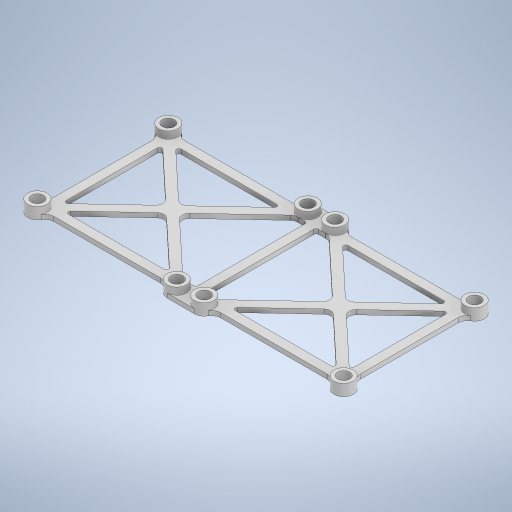
# Autodesk Inventor part: Display_Standof_2.5
Saved by Autodesk Inventor 2023 (Build 270158000, 158)
## iProperties
Created: 2023-02-18
Part Number: Display_Standof_2.5
Material: Generisch
Document SubType Name: Modeling
Designer: dvd62
Density: 1 g/cm^3
Appearance: Vorgabe
Author: dvd62
Autodesk Inventor part; units mm, degrees
ref_plane "YZ Plane" through (0, 0, 0) normal (1, 0, 0) x (0, 1, 0)
ref_plane "XZ Plane" through (0, 0, 0) normal (0, 1, 0) x (-1, 0, 0)
ref_plane "XY Plane" through (0, 0, 0) normal (0, 0, 1) x (1, 0, 0)
sketch "Skizze1" plane through (0, 0, 0) normal (0, 1, 0) x (-1, 0, 0)
  circle A0 centre (0, 0) radius 1.35
  circle A1 centre (-30.8, 0) radius 1.35
  circle A2 centre (-36.83, 0) radius 1.35
  circle A3 centre (-67.63, 0) radius 1.35
  circle A4 centre (0, -28.9) radius 1.35
  circle A5 centre (-30.8, -28.9) radius 1.35
  circle A6 centre (-36.83, -28.9) radius 1.35
  circle A7 centre (-67.63, -28.9) radius 1.35
  line L0 (0, 0) -> (-67.63, 0) construction
  line L1 (-67.63, 0) -> (-67.63, -28.9) construction
  line L2 (-67.63, -28.9) -> (0, -28.9) construction
  line L3 (0, -28.9) -> (0, 0) construction
  circle A8 centre (0, -28.9) radius 2.15
  circle A9 centre (-30.8, -28.9) radius 2.15
  circle A10 centre (-36.83, -28.9) radius 2.15
  circle A11 centre (-67.63, -28.9) radius 2.15
  circle A12 centre (-67.63, 0) radius 2.15
  circle A13 centre (-36.83, 0) radius 2.15
  circle A14 centre (-30.8, 0) radius 2.15
  circle A15 centre (0, 0) radius 2.15
  line L4 (0, -26.75) -> (0, -2.15)
  line L5 (-2.15, 0) -> (-28.65, 0)
  line L6 (-32.95, 0) -> (-34.68, 0)
  line L7 (-38.98, 0) -> (-65.48, 0)
  line L8 (-67.63, -2.15) -> (-67.63, -26.75)
  line L9 (-65.48, -28.9) -> (-38.98, -28.9)
  line L10 (-34.68, -28.9) -> (-32.95, -28.9)
  line L11 (-28.65, -28.9) -> (-2.15, -28.9)
  line L12 (-2, -2) -> (-65.63, -2)
  line L13 (-65.63, -2) -> (-65.63, -26.9)
  line L14 (-65.63, -26.9) -> (-2, -26.9)
  line L15 (-2, -26.9) -> (-2, -2)
  line L16 (0, -28.9) -> (-30.8, 0) construction
  line L17 (0, 0) -> (-30.8, -28.9) construction
  line L18 (-36.83, -28.9) -> (-67.63, 0) construction
  line L19 (-67.63, -28.9) -> (-36.83, 0) construction
  line L20 (-27.2071, -2) -> (-2, -25.6521)
  line L21 (-3.5929, -26.9) -> (-30.0963, -2.0316)
  line L22 (-2, -3.2479) -> (-27.2071, -26.9)
  line L23 (-3.5929, -2) -> (-30.0963, -26.8684)
  line L24 (-64.0371, -2) -> (-37.5337, -26.8684)
  line L25 (-65.63, -3.2479) -> (-40.4229, -26.9)
  line L26 (-37.5337, -2.0316) -> (-64.0371, -26.9)
  line L27 (-65.63, -25.6521) -> (-40.4229, -2)
  line L28 (-33.815, -2) -> (-33.815, -26.9) construction
  line L29 (-32.815, -26.9) -> (-32.815, -2)
  line L30 (-34.815, -2) -> (-34.815, -26.9)
  line L31 (-36.83, -31.05) -> (-30.8, -31.05)
  line L32 (-30.8, -26.75) -> (-36.83, -26.75)
  line L33 (-30.8, -2.15) -> (-36.83, -2.15)
  line L34 (-30.8, 2.15) -> (-36.83, 2.15)
  point P0 (-31.589, -2)
  point P1 (-16.8614, -14.45)
  point P2 (-31.589, -26.9)
  point P3 (-36.041, -26.9)
  point P4 (-50.7686, -14.45)
  point P5 (-36.041, -2)
  point P6 (-52.23, -13.0787)
  point P7 (-53.6914, -14.45)
  point P8 (-52.23, -15.8213)
  point P9 (-13.9386, -14.45)
  point P10 (-15.4, -13.0787)
  point P11 (-15.4, -15.8213)
  point P12 (-34.815, -2.15)
  point P13 (-32.815, -2.15)
  point P14 (-32.815, -26.75)
  point P15 (-34.815, -26.75)
  dimension "d0" = 2.7
  dimension "d1" = 2.7
  dimension "d2" = 2.7
  dimension "d3" = 2.7
  dimension "d4" = 2.7
  dimension "d5" = 2.7
  dimension "d7" = 2.7
  dimension "d8" = 2.7
  dimension "d9" = 30.8
  dimension "d10" = 6.03
  dimension "d11" = 30.8
  dimension "d12" = 28.9
  dimension "d13" = 30.8
  dimension "d14" = 6.03
  dimension "d15" = 30.8
  dimension "d16" = 0.8
  dimension "d17" = 0.8
  dimension "d18" = 0.8
  dimension "d19" = 0.8
  dimension "d20" = 0.8
  dimension "d21" = 0.8
  dimension "d22" = 0.8
  dimension "d23" = 0.8
  dimension "d24" = 2
  dimension "d25" = 2
  dimension "d26" = 2
  dimension "d27" = 2
  dimension "d28" = 2
  dimension "d29" = 2
  dimension "d30" = 2
  dimension "d31" = 2
  dimension "d34" = 2
  constraints: 62 end point, 28 point on circle, 16 centre point, 9 point on line, 8 parallel, 6 tangent, 4 vertical, 2 coincident, 1 horizontal, 49 other
  measures "d0" diameter of A0
  measures "d1" diameter of A1
  measures "d2" diameter of A2
  measures "d3" diameter of A3
  measures "d4" diameter of A4
  measures "d5" diameter of A5
  measures "d7" diameter of A6
  measures "d8" diameter of A7
  measures "d9" distance of L16.end point (0, 0)
  measures "d10" distance of A2.centre L16.end
  measures "d11" distance of A3.centre A2.centre
  measures "d12" distance of L3.start point (0, 0)
  measures "d13" distance of L17.end A4.centre
  measures "d14" distance of L17.end L18.start
  measures "d15" distance of L1.end L18.start
  measures "d16" radial gap between concentric circles of A4 A8
  measures "d17" radial gap between concentric circles of A5 A9
  measures "d18" radial gap between concentric circles of A6 A10
  measures "d19" radial gap between concentric circles of A7 A11
  measures "d20" radial gap between concentric circles of A3 A12
  measures "d21" radial gap between concentric circles of A2 A13
  measures "d22" radial gap between concentric circles of A1 A14
  measures "d23" radial gap between concentric circles of A0 A15
  measures "d24" distance between parallel lines of L3 L15
  measures "d26" distance between parallel lines of L8 L13
  measures "d28" distance between parallel lines of L21 L20
  measures "d29" distance between parallel lines of L22 L23
  measures "d30" distance between parallel lines of L25 L24
  measures "d31" distance between parallel lines of L26 L27
  measures "d34" distance between parallel lines of L29 L30
extrude "Extrusion1" add sketch "Skizze1" along normal blind 1 contours A8 | A8 L11 A9 L14 L15 L12 A14 L5 A15 L4 | A15 | A9 L14 | L31 A10 L10 A9 | L14 A9 | A9 L23 L21 L22 L14 | A14 L12 | L10 A10 L14 A9 | A10 L14 | L14 L29 L32 A9 | A14 L6 A13 L34 | L12 L20 L23 L21 A14 | A14 L12 | L9 A11 L8 A12 L7 A13 L12 L13 L14 A10 | L23 L20 L22 L21 | L14 L30 L32 L29 | L21 L22 L20 L15 L14 | A14 L12 A13 L6 | A13 L12 | A14 L33 L29 L12 | L14 A10 | A10 L32 L30 L14 | L14 L25 L26 L24 A10 | A11 | L32 L30 L33 L29 | L23 L12 L15 L22 L20 | L29 L33 L30 L12 | L12 L30 L33 A13 | A13 L12 | A13 L26 L24 L27 L12 | A12 | L26 L25 L27 L24 | L14 L13 L27 L25 L26 | L27 L25 L13 L12 L24
sketch "Skizze2" plane through (0, 1, 0) normal (0, 1, 0) x (1, 0, 0)
  circle A0 centre (0, 28.9) radius 1.35 projected
  arc A1 (2.15, 28.9) -> (0, 26.75) centre (0, 28.9) ccw projected
  arc A2 (38.98, 0) -> (28.65, 28.9) centre (30.8, 28.9) ccw projected
  circle A3 centre (30.8, 28.9) radius 1.35 projected
  circle A4 centre (36.83, 28.9) radius 1.35 projected
  arc A5 (38.98, 28.9) -> (38.98, 0) centre (36.83, 28.9) ccw projected
  arc A6 (67.63, 26.75) -> (65.48, 28.9) centre (67.63, 28.9) ccw projected
  circle A7 centre (67.63, 28.9) radius 1.35 projected
  circle A8 centre (67.63, 0) radius 1.35 projected
  arc A9 (65.48, 0) -> (67.63, 2.15) centre (67.63, 0) ccw projected
  arc A10 (38.98, 0) -> (38.98, 0) centre (36.83, 0) ccw projected
  arc A11 (28.65, 0) -> (38.98, 0) centre (30.8, 0) ccw projected
  circle A12 centre (30.8, 0) radius 1.35 projected
  arc A13 (0, 2.15) -> (2.15, 0) centre (0, 0) ccw projected
  circle A14 centre (0, 0) radius 1.35 projected
  arc A15 (36.83, -2.15) -> (38.98, 0) centre (36.83, 0) ccw projected
  line L0 (38.98, 0) -> (65.48, 0) projected
  arc A16 (65.48, 0) -> (67.63, 2.15) centre (67.63, 0) ccw projected
  line L1 (67.63, 2.15) -> (67.63, 26.75) projected
  arc A17 (67.63, 26.75) -> (65.48, 28.9) centre (67.63, 28.9) ccw projected
  line L2 (65.48, 28.9) -> (38.98, 28.9) projected
  arc A18 (38.98, 28.9) -> (36.83, 31.05) centre (36.83, 28.9) ccw projected
  arc A19 (30.8, 31.05) -> (28.65, 28.9) centre (30.8, 28.9) ccw projected
  line L3 (28.65, 28.9) -> (2.15, 28.9) projected
  arc A20 (2.15, 28.9) -> (0, 26.75) centre (0, 28.9) ccw projected
  line L4 (0, 26.75) -> (0, 2.15) projected
  arc A21 (0, 2.15) -> (2.15, 0) centre (0, 0) ccw projected
  line L5 (2.15, 0) -> (28.65, 0) projected
  arc A22 (28.65, 0) -> (30.8, -2.15) centre (30.8, 0) ccw projected
  line L6 (32.815, 26.75) -> (32.815, 2.15) projected
  arc A23 (30.8, 2.15) -> (30.0963, 2.0316) centre (30.8, 0) ccw projected
  line L7 (30.0963, 2.0316) -> (16.8614, 14.45) projected
  line L8 (16.8614, 14.45) -> (30.0963, 26.8684) projected
  arc A24 (30.0963, 26.8684) -> (30.8, 26.75) centre (30.8, 28.9) ccw projected
  circle A25 centre (67.63, 0) radius 1.35 projected
  circle A26 centre (67.63, 28.9) radius 1.35 projected
  circle A27 centre (36.83, 28.9) radius 1.35 projected
  line L9 (64.0371, 2) -> (40.4229, 2) projected
  line L10 (40.4229, 2) -> (52.23, 13.0787) projected
  line L11 (52.23, 13.0787) -> (64.0371, 2) projected
  line L12 (65.63, 3.2479) -> (53.6914, 14.45) projected
  line L13 (53.6914, 14.45) -> (65.63, 25.6521) projected
  line L14 (65.63, 25.6521) -> (65.63, 3.2479) projected
  line L15 (40.4229, 26.9) -> (64.0371, 26.9) projected
  line L16 (64.0371, 26.9) -> (52.23, 15.8213) projected
  line L17 (52.23, 15.8213) -> (40.4229, 26.9) projected
  circle A28 centre (0, 0) radius 1.35 projected
  line L18 (2, 25.6521) -> (13.9386, 14.45) projected
  line L19 (13.9386, 14.45) -> (2, 3.2479) projected
  line L20 (2, 3.2479) -> (2, 25.6521) projected
  line L21 (3.5929, 2) -> (15.4, 13.0787) projected
  line L22 (15.4, 13.0787) -> (27.2071, 2) projected
  line L23 (27.2071, 2) -> (3.5929, 2) projected
  line L24 (3.5929, 26.9) -> (27.2071, 26.9) projected
  line L25 (27.2071, 26.9) -> (15.4, 15.8213) projected
  line L26 (15.4, 15.8213) -> (3.5929, 26.9) projected
  circle A29 centre (0, 28.9) radius 1.35 projected
  circle A30 centre (30.8, 28.9) radius 1.35 projected
  circle A31 centre (36.83, 0) radius 1.35 projected
  circle A32 centre (30.8, 0) radius 1.35 projected
  arc A33 (36.83, 26.75) -> (37.5337, 26.8684) centre (36.83, 28.9) ccw projected
  line L27 (37.5337, 26.8684) -> (50.7686, 14.45) projected
  line L28 (50.7686, 14.45) -> (37.5337, 2.0316) projected
  arc A34 (37.5337, 2.0316) -> (36.83, 2.15) centre (36.83, 0) ccw projected
  line L29 (34.815, 2.15) -> (34.815, 26.75) projected
  circle A35 centre (0, 28.9) radius 1.35
  circle A36 centre (0, 28.9) radius 1.35 projected
  circle A37 centre (0, 28.9) radius 2.15
  circle A38 centre (30.8, 28.9) radius 1.35 projected
  circle A39 centre (30.8, 28.9) radius 2.15
  circle A40 centre (30.8, 28.9) radius 1.35
  circle A41 centre (36.83, 28.9) radius 1.35 projected
  circle A42 centre (36.83, 28.9) radius 1.35
  circle A43 centre (36.83, 28.9) radius 2.15
  circle A44 centre (67.63, 28.9) radius 1.35
  circle A45 centre (67.63, 28.9) radius 2.15
  circle A46 centre (67.63, 0) radius 1.35
  circle A47 centre (67.63, 0) radius 2.15
  circle A48 centre (36.83, 0) radius 1.35
  circle A49 centre (36.83, 0) radius 1.35 projected
  circle A50 centre (30.8, 0) radius 1.35
  circle A51 centre (30.8, 0) radius 2.15
  circle A52 centre (0, 0) radius 1.35
  circle A53 centre (0, 0) radius 2.15
  line L30 (36.83, 31.05) -> (30.8, 31.05) projected
  line L31 (30.8, -2.15) -> (36.83, -2.15) projected
  line L32 (32.815, 2.15) -> (30.8, 2.15) projected
  line L33 (30.8, 26.75) -> (32.815, 26.75) projected
  line L34 (34.815, 26.75) -> (36.83, 26.75) projected
  line L35 (36.83, 2.15) -> (34.815, 2.15) projected
  circle A54 centre (36.83, 0) radius 1.35 projected
  circle A55 centre (36.83, 0) radius 2.15
  point P0 (33.15, 28.9)
  point P1 (34.48, 28.9)
  point P2 (65.48, 0)
  point P3 (36.9895, 26.7559)
  point P4 (36.83, 26.75)
  point P5 (37.5337, 26.8684)
  point P6 (38.98, 28.9)
  point P7 (30.0963, 26.8684)
  point P8 (30.8, 26.75)
  point P9 (32.95, 28.9)
  point P10 (30.0963, 2.0316)
  point P11 (28.65, 0)
  point P12 (32.95, 0)
  point P13 (30.8, 2.15)
  point P14 (2.15, 0)
  point P15 (0, 2.15)
  point P16 (0, 26.75)
  point P17 (2.15, 28.9)
  point P18 (38.98, 0)
  point P19 (37.5337, 2.0316)
  point P20 (36.83, -2.15)
  constraints: 16 centre point, 16 coincident, 13 concentric, 3 other
extrude "Extrusion2" add sketch "Skizze2" along normal blind 1.54 contours A37 A1 | A53 A13 | A19 A2 | A2 A19 A5 A39 A24 | A11 A10 A5 A31 | A5 A31 A10 | A10 A11 | A19 A39 A5 | A47 A9 | A22 A11 A5 | A5 A11 A22 | A51 A23 A5 A11 | A11 A5 A51 | A43 A18 A5 A4 | A5 A4 A43 A33 | A45 A6
fillet "Rundung1" radius 0.5 16 edges at (2, 0.5, -25.6521) (3.5929, 0.5, -26.9) (3.5929, 0.5, -2) (2, 0.5, -3.2479) (27.2071, 0.5, -2) (27.2071, 0.5, -26.9) (40.4229, 0.5, -26.9) (40.4229, 0.5, -2) (64.0371, 0.5, -26.9) (64.0371, 0.5, -2) (65.63, 0.5, -3.2479) (65.63, 0.5, -25.6521) (32.815, 0.5, -2.15) (34.815, 0.5, -2.15) (32.815, 0.5, -26.75) (34.815, 0.5, -26.75)
fillet "Rundung1" radius 1.5 12 edges at (13.9386, 0.5, -14.45) (15.4, 0.5, -13.0787) (16.8614, 0.5, -14.45) (15.4, 0.5, -15.8213) (50.7686, 0.5, -14.45) (52.23, 0.5, -13.0787) (53.6914, 0.5, -14.45) (52.23, 0.5, -15.8213) (37.5337, 0.5, -2.0316) (37.5337, 0.5, -26.8684) (30.0963, 0.5, -26.8684) (30.0963, 0.5, -2.0316)
fillet "Rundung1" radius 2 12 edges at (2.15, 0.5, 0) (0, 0.5, -2.15) (0, 0.5, -26.75) (2.15, 0.5, -28.9) (28.65, 0.5, -28.9) (28.65, 0.5, 0) (38.98, 0.5, -28.9) (38.98, 0.5, 0) (67.63, 0.5, -2.15) (67.63, 0.5, -26.75) (65.48, 0.5, -28.9) (65.48, 0.5, 0)
equation "\"d0\" = holeDim"
equation "\"d1\" = holeDim"
equation "\"d2\" = holeDim"
equation "\"d3\" = holeDim"
equation "\"d4\" = holeDim"
equation "\"d5\" = holeDim"
equation "\"d7\" = holeDim"
equation "\"d8\" = holeDim"
equation "\"d11\" = d9"
equation "\"d13\" = d9"
equation "\"d14\" = d10"
equation "\"d16\" = spacerThick"
equation "\"d17\" = spacerThick"
equation "\"d18\" = spacerThick"
equation "\"d19\" = spacerThick"
equation "\"d20\" = spacerThick"
equation "\"d21\" = spacerThick"
equation "\"d22\" = spacerThick"
equation "\"d23\" = spacerThick"
equation "\"d24\" = clearanceThick"
equation "\"d25\" = clearanceThick"
equation "\"d26\" = clearanceThick"
equation "\"d27\" = clearanceThick"
equation "\"d28\" = clearanceThick"
equation "\"d29\" = clearanceThick"
equation "\"d30\" = clearanceThick"
equation "\"d31\" = clearanceThick"
equation "\"holeDim\" = 2.7"
equation "\"spacerHight\" = 1.54"
equation "\"clearanHight\" = 1"
equation "\"spacerThick\" = 0.8"
equation "\"clearanceThick\" = 2"
